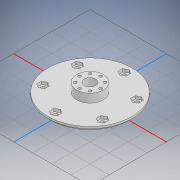
# Autodesk Inventor part: 000.005.001.003 - Вал
Saved by Autodesk Inventor 2022 (Build 260153000, 153)
## iProperties
Created: 2022-11-17
Part Number: 000.005.001.003 - Вал
Material: Типовые
Document SubType Name: Modeling
Designer: Petrov Ivan
Density: 1 g/cm^3
Appearance: По умолчанию
Author: Petrov Ivan
Autodesk Inventor part; units mm, degrees
ref_plane "YZ Plane" through (0, 0, 0) normal (1, 0, 0) x (0, 1, 0)
ref_plane "XZ Plane" through (0, 0, 0) normal (0, 1, 0) x (-1, 0, 0)
ref_plane "XY Plane" through (0, 0, 0) normal (0, 0, 1) x (1, 0, 0)
sketch "Эскиз1" plane through (0, 0, 0) normal (0, 1, 0) x (-1, 0, 0)
  circle A0 centre (0, 0) radius 44
  dimension "d0" = 88
  constraints: 1 centre point, 1 coincident
  measures "d0" diameter of A0
extrude "Выдавливание1" add sketch "Эскиз1" along normal blind 5
sketch "Эскиз2" plane through (0, 5, 0) normal (0, 1, 0) x (1, 0, 0)
  circle A0 centre (0, 0) radius 14
  dimension "d3" = 28
  constraints: 1 centre point, 1 coincident
  measures "d3" diameter of A0
extrude "Выдавливание2" add sketch "Эскиз2" along normal blind 9
sketch "Эскиз3" plane through (0, 14, 0) normal (0, 1, 0) x (1, 0, 0)
  circle A0 centre (0, 0) radius 6
  dimension "d6" = 12
  constraints: 1 centre point, 1 coincident
  measures "d6" diameter of A0
extrude "Выдавливание3" cut sketch "Эскиз3" against normal through all
sketch "Эскиз4" plane through (0, 5, 0) normal (0, 1, 0) x (1, 0, 0)
  circle A0 centre (0, -36) radius 2.5
  point P0 (0, 0)
  dimension "d9" = 5
  dimension "d10" = 36
  constraints: 1 centre point, 1 vertical alignment
  measures "d9" diameter of A0
  measures "d10" distance of A0.centre point (0, 0)
extrude "Выдавливание4" cut sketch "Эскиз4" against normal through all
pattern_circular "Круговой массив1" count 6 over 360 about axis through (0, 5, 0) along (0, 1, 0) of "Выдавливание4"
sketch "Эскиз5" plane through (0, 14, 0) normal (0, 1, 0) x (1, 0, 0)
  circle A0 centre (0, 0) radius 14
  circle A1 centre (-11, 0) radius 1.2813
  circle A2 centre (-7.7782, -7.7782) radius 1.2813
  circle A3 centre (0, -11) radius 1.2813
  circle A4 centre (7.7782, -7.7782) radius 1.2813
  circle A5 centre (11, 0) radius 1.2813
  circle A6 centre (7.7782, 7.7782) radius 1.2813
  circle A7 centre (0, 11) radius 1.2813
  circle A8 centre (-7.7782, 7.7782) radius 1.2813
  constraints: 9 centre point
extrude "Выдавливание5" cut sketch "Эскиз5" against normal through all contours A1 | A2 | A3 | A4 | A5 | A6 | A7 | A8
offset faces "Размер1" outward -0.25 faces at (9.0553, 4.6667, 7.8813) (-6.5011, 4.6667, 7.8813) (1.2771, 4.6667, 11.1031) (-9.7229, 4.6667, 0.1031) (-6.5011, 4.6667, -7.6751) (1.2771, 4.6667, -10.8969) (9.0553, 4.6667, -7.6751) (12.2771, 4.6667, 0.1031)
sketch "Эскиз6" plane through (0, 0, 0) normal (0, -1, 0) x (1, 0, 0)
  circle A0 centre (11, 0) radius 1.5312 projected
  circle A1 centre (11, 0) radius 2.5
  point P0 (0, 0)
  dimension "d19" = 5
  constraints: 1 centre point, 1 coincident
  measures "d19" diameter of A1
extrude "Выдавливание6" cut sketch "Эскиз6" against normal blind 5.5
pattern_circular "Круговой массив2" count 8 over 360 about axis through (0, 14, 0) along (0, -1, 0) of "Выдавливание6"
sketch "Эскиз7" plane through (0, 5, 0) normal (0, 1, 0) x (1, 0, 0)
  circle A0 centre (-31.1769, 18) radius 2.5 projected
  line L0 (-31.1769, 22.9075) -> (-26.9269, 20.4537)
  line L1 (-26.9269, 20.4537) -> (-26.9269, 15.5463)
  line L2 (-26.9269, 15.5463) -> (-31.1769, 13.0925)
  line L3 (-31.1769, 13.0925) -> (-35.4269, 15.5463)
  line L4 (-35.4269, 15.5463) -> (-35.4269, 20.4537)
  line L5 (-35.4269, 20.4537) -> (-31.1769, 22.9075)
  circle A1 centre (-31.1769, 18) radius 8.0069
  point P0 (0, 0)
  dimension "d25" = 8.5
  constraints: 12 end point, 2 coincident, 1 centre point, 13 other
  measures "d25" distance between parallel lines of L1 L4
extrude "Выдавливание7" cut sketch "Эскиз7" against normal blind 3 contours A0 | L0 L1 L2 L3 L4 L5
pattern_circular "Круговой массив3" count 6 over 360 about axis through (0, 5, 0) along (0, 1, 0) of "Выдавливание7"
chamfer "Фаска1" distance 3 angle 45 1 edges at (44, 0, 0)
